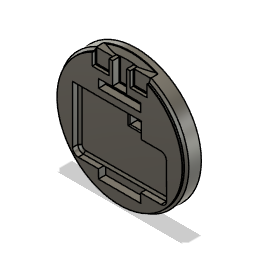
chamber top (Autodesk Fusion 360 design; units mm, degrees)
Autodesk Fusion 360 part; units mm, degrees
sketch "base" plane through (0, 0, 0) normal (0, 0, 1) x (1, 0, 0)
  circle A0 centre (0, 0) radius 46.25
  circle A1 centre (0, 0) radius 43.85
  circle A2 centre (0, 0) radius 41.85
  dimension "d3" = 92.5
  dimension "d6" = 87.7
  dimension "d19" = 83.7
  constraint coincident A0.centre A1.centre
  constraint concentric A1 A2
  measures "d3" diameter of A0
  measures "d6" diameter of A1
  measures "d19" diameter of A2
sketch "wire hole" plane through (0, 0, 0) normal (0, 0, 1) x (1, 0, 0)
  line L0 (1.4953, 2.9941) -> (12.4953, 2.9941)
  line L1 (1.4953, 2.9941) -> (1.4953, 11.9941)
  line L2 (1.4953, 11.9941) -> (12.4953, 11.9941)
  line L3 (12.4953, 2.9941) -> (12.4953, 11.9941)
  line L4 (43.2544, 6.8774) -> (45.6908, 6.8152)
  line L5 (45.6908, 6.8152) -> (43.5237, 4.9071)
  line L6 (43.5237, 4.9071) -> (43.2544, 6.8774)
sketch "components" plane through (0, 0, 0) normal (0, 0, 1) x (1, 0, 0)
  line L0 (-14.9999, 26) -> (15.0001, 26)
  line L1 (15.0001, 26) -> (15.0001, 20)
  line L2 (15.0001, 20) -> (-14.9999, 20)
  line L3 (-14.9999, 20) -> (-14.9999, 26)
  line L4 (15.0001, -36) -> (-14.9999, -36)
  line L5 (-33.4999, 3) -> (-43.2989, 3)
  line L6 (-43.2989, 3) -> (-43.1087, 5.0432)
  line L7 (-43.1087, 5.0432) -> (-42.8221, 7.0752)
  line L8 (-42.8221, 7.0752) -> (-42.4398, 9.0913)
  line L9 (-42.4398, 9.0913) -> (-41.9627, 11.0871)
  line L10 (-41.9627, 11.0871) -> (-41.3917, 13.0582)
  line L11 (-41.3917, 13.0582) -> (-40.7283, 15)
  line L12 (-40.7283, 15) -> (15.5011, 15)
  line L13 (15.5011, 15) -> (15.5011, 3.5567)
  line L14 (-7.4999, 42) -> (-7.4999, 31.4649)
  line L15 (-7.4999, 31.4649) -> (-19.4999, 31.4649)
  line L16 (19.5001, 31.4649) -> (7.5001, 31.4649)
  line L17 (7.5001, 31.4649) -> (7.5001, 42)
  line L18 (7.5001, 42) -> (5.0001, 42)
  line L19 (5.0001, 42) -> (5.0001, 26.3188)
  line L20 (5.0001, 26.3188) -> (-4.9999, 26.3188)
  line L21 (-4.9999, 26.3188) -> (-4.9999, 42)
  line L22 (-4.9999, 42) -> (-7.4999, 42)
  line L23 (29.5002, -29.4433) -> (-29.4783, -29.7485)
  line L24 (-33.499, -25.7485) -> (-33.499, 15)
  line L25 (33.4794, -25.4227) -> (33.35, -0.4069)
  line L26 (29.3455, 3.5724) -> (15.5011, 3.5567)
  arc A0 (33.35, -0.4069) -> (29.3455, 3.5724) centre (29.3501, -0.4276) ccw
  arc A1 (29.5002, -29.4433) -> (33.4794, -25.4227) centre (29.4795, -25.4434) ccw
  arc A2 (-33.499, -25.7485) -> (-29.4783, -29.7485) centre (-29.499, -25.7485) ccw
  circle A3 centre (0, 0) radius 44.6
  line L27 (19.5001, 31.4649) -> (19.5001, 41.9999)
  line L28 (-19.4999, 31.4649) -> (-19.4999, 41.9999)
  line L29 (19.5001, 41.9999) -> (-19.4999, 41.9999)
  arc A4 (19.5001, 41.9999) -> (-19.4999, 41.9999) centre (0.0001, 0.0293) ccw
  line L30 (-14.9999, -36) -> (-15.0326, -29.6737)
  line L31 (15.0001, -36) -> (14.9666, -29.5185)
  point P0 (33.5001, -29.4226)
  point P1 (-33.499, -29.7693)
  point P2 (33.3294, 3.5769)
  point P3 (0, 44.6)
  point P4 (0, 44.6)
  dimension "d36" = 67
  dimension "d37" = 33
  dimension "d40" = 4
  dimension "d41" = 89.2
  dimension "d42" = 10.535
  dimension "d43" = 10.535
  constraint coincident L12 L24.end
  constraint perpendicular L12 L24
  constraint perpendicular L23 L25
  constraint coincident L13.end L26.end
  constraint coincident P2 L25
  constraint coincident P2 L26
  constraint tangent L25 A0
  constraint tangent L26 A0
  constraint coincident P0 L23
  constraint coincident P0 L25
  constraint tangent L23 A1
  constraint tangent L25 A1
  constraint coincident P1 L23
  constraint coincident P1 L24
  constraint tangent L23 A2
  constraint tangent L24 A2
  constraint coincident A3.centre origin
  constraint coincident L16.start L27.start
  constraint perpendicular L16 L27
  constraint coincident L15.end L28.start
  constraint perpendicular L15 L28
  constraint coincident A3 P4
  constraint coincident L4.end L30.start
  constraint coincident L23 L30.end
  constraint perpendicular L23 L30
  constraint coincident L4.start L31.start
  constraint coincident L23 L31.end
  constraint perpendicular L23 L31
  measures "d36" distance of P0 P1
  measures "d37" distance of P0 P2
  measures "d40" radius of A2
  measures "d41" diameter of A3
  measures "d42" distance of L16.start L27.end
  measures "d43" distance of L15.end L28.end
extrude "Extrude11" add sketch "components" along normal blind 1.5 and the other way blind 7.5 contours L0 L1 L2 L3 | L4 L23 L30 L31 | L12 L13 L23 L24 L25 L26 A0 A1 A2 | L5 L6 L7 L8 L9 L10 L11 L12 L24 | L14 L15 L16 L17 L18 L19 L20 L21 L22 A3 L27 L28 L29 | L14 L15 A3 L28 L29 | L19 L20 L21 L29 | L16 L17 A3 L27 L29
sketch "ring" plane through (0, 0, 0) normal (1, 0, 0) x (0, 0, -1)
  line L0 (0, 44.6) -> (-0.5928, 44.6924) construction
  circle A0 centre (-0.5928, 44.6924) radius 0.5
  point P0 (0, 44.6)
  dimension "d52" = 0.6
  dimension "d53" = 1
  constraint coincident P0 L0.start
  constraint coincident L0.end A0.centre
  measures "d52" distance of P0 L0.end
  measures "d53" diameter of A0
revolve "Revolve1" cut sketch "ring" angle 360 about axis through (0, 0, 1.75) along (0, 0, 1)
fillet "Fillet1" [suppressed]
extrude "Extrude12" add sketch "base" against normal blind 7.5 contours A0
chamfer "Chamfer1" distance 1.6 angle 45 1 edges at (-43.1201, -16.7247, 0)
extrude "Extrude13" cut sketch "components" against normal blind 5.25 from surface at 1.5 contours L12 L13 L23 L24 L25 L26 A0 A1 A2
chamfer "Chamfer2" distance 1.5 angle 45 1 faces at (-17.1656, -2.3973, -3.75)
extrude "Extrude14" cut sketch "components" against normal blind 5.1 from surface at 1.5 contours L0 L1 L2 L3 | L4 L23 L30 L31
extrude "Extrude15" cut sketch "components" against normal blind 2.7 from surface at 1.5 contours L14 L15 A3 L28 L29 | A3 L28 L29 | A3 L27 L29 | L16 L17 A3 L27 L29
extrude "Extrude16" cut sketch "components" against normal blind 5.1 from surface at 1.5 contours L19 L20 L21 L29
extrude "Extrude18" add sketch "components" against normal blind 7.5 contours L18 L22 A3 L29
extrude "Extrude17" cut sketch "components" against normal blind 5.1 from surface at 1.5 contours L18 L22 A3 L29 | A3 L29 A4
chamfer "Chamfer4" distance 3.5 angle 45 1 edges at (0, 46.25, -3.6)
chamfer "Chamfer5" distance 0.5 angle 45 3 edges at (-7.4999, 36.7324, -1.2) (-13.4999, 31.4649, -1.2) (-19.4999, 36.4808, -1.2)
chamfer "Chamfer6" distance 0.5 angle 45 3 edges at (7.5001, 36.7324, -1.2) (13.5001, 31.4649, -1.2) (19.5001, 36.4807, -1.2)
chamfer "Chamfer7" distance 0.5 angle 45 3 edges at (5.0001, 34.1594, -3.6) (0.0001, 26.3188, -3.6) (-4.9999, 34.1594, -3.6)
extrude "Extrude19" add sketch "base" along normal blind 4 from surface at -10.5
extrude "Extrude20" cut sketch "wire hole" against normal blind 13 contours L0 L1 L2 L3
fillet "Fillet2" radius 0.75 4 edges at (6.9953, 2.9941, -10.5) (6.9953, 11.9941, -10.5) (1.4953, 7.4941, -10.5) (12.4953, 7.4941, -10.5)
fillet "Fillet3" radius 0.75 4 edges at (6.9953, 2.9941, -3.75) (12.4953, 7.4941, -3.75) (6.9953, 11.9941, -3.75) (1.4953, 7.4941, -3.75)
fillet "Fillet4" radius 0.6 1 edges at (-0.0001, -44.6, 1.0842)
equation "d3 = ChamberSize"
equation "d6 = ChamberSize - ChamberOffset"
equation "ChamberLip = 4 mm"
equation "ChamberSize = 92.5 mm"
equation "ChamberOffset = 4.8 mm"
equation "ChamberInner = 4 mm"
equation "ChamberHeight = 40 mm"
equation "d19 = ChamberSize - ChamberOffset - ChamberInner"
equation "d46 = TopRaise"
equation "d52 = RingOffset"
equation "d53 = RingSize"
equation "d60 = ComponentHeight - TopRaise"
equation "TopRaise = 1.5 mm"
equation "MainComponent = 5.25 mm"
equation "Expansion = 5.10 mm"
equation "USB = 2.7 mm"
equation "Jack = 5.1 mm"
equation "d67 = -MainComponent"
equation "d72 = -Expansion"
equation "d77 = TopRaise"
equation "d78 = -USB"
equation "d80 = TopRaise"
equation "d81 = TopRaise"
equation "d82 = TopRaise"
equation "d83 = -Jack"
equation "d85 = TopRaise"
equation "d86 = -Jack"
equation "d88 = -ComponentHeight + TopRaise"
equation "ComponentHeight = 9 mm"
equation "d95 = -ComponentHeight - TopRaise"
equation "d96 = ChamberLip"
equation "d98 = -ComponentHeight - ChamberLip"
equation "RingOffset = 0.6 mm"
equation "RingSize = 1 mm"
named bodies: "chamber top"
